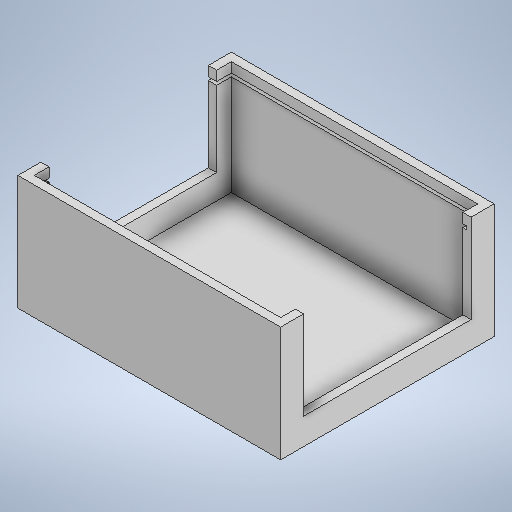
# Autodesk Inventor part: 3 Pzem test
Saved by Autodesk Inventor 2025.3 (Build 293356000, 356)
## iProperties
Created: 2026-02-05
Part Number: 3 Pzem test
Material: Generic
Document SubType Name: Modeling
Designer: Maulana
Density: 1 g/cm^3
Appearance: Default
Author: Maulana
Autodesk Inventor part; units mm, degrees
ref_plane "YZ Plane" through (0, 0, 0) normal (1, 0, 0) x (0, 1, 0)
ref_plane "XZ Plane" through (0, 0, 0) normal (0, 1, 0) x (-1, 0, 0)
sketch "Sketch1" plane through (0, 0, 0) normal (0, 1, 0) x (-1, 0, 0)
  line L0 (37.5, 30) -> (-37.5, 30)
  line L1 (-37.5, 30) -> (-37.5, -30)
  line L2 (-37.5, -30) -> (37.5, -30)
  line L3 (37.5, -30) -> (37.5, 30)
  line L4 (37.5, 30) -> (-37.5, -30) construction
  line L5 (-37.5, 30) -> (37.5, -30) construction
  line L6 (38, 30.5) -> (-38, 30.5)
  line L7 (-38, 30.5) -> (-38, -30.5)
  line L8 (-38, -30.5) -> (38, -30.5)
  line L9 (38, -30.5) -> (38, 30.5)
  line L10 (38, 30.5) -> (-38, -30.5) construction
  line L11 (-38, 30.5) -> (38, -30.5) construction
  point P0 (0, 0)
  dimension "d0" = 75
  dimension "d1" = 60
  dimension "d2" = 76
  dimension "d3" = 61
  constraints: 24 end point, 4 midpoint, 4 parallel, 2 horizontal, 2 perpendicular
  measures "d0" distance of L2.end L1.end
  measures "d1" distance of L1.end L0.end
  measures "d2" distance of L8.end L7.end
  measures "d3" distance of L7.end L6.end
extrude "Extrusion1" add sketch "Sketch1" along normal blind 35
sketch "Sketch2" plane through (0, 0, 0) normal (0, -1, 0) x (1, 0, 0)
  line L0 (37.5, -30) -> (37.5, 30) projected
  line L1 (-37.5, 30) -> (37.5, 30)
  line L2 (37.5, 30) -> (37.5, -30)
  line L3 (37.5, -30) -> (-37.5, -30)
  line L4 (-37.5, -30) -> (-37.5, 30)
  line L5 (-37.5, 30) -> (37.5, -30) construction
  line L6 (37.5, 30) -> (-37.5, -30) construction
  point P0 (0, 0)
  constraints: 12 end point, 2 midpoint, 2 parallel, 1 horizontal, 1 perpendicular
extrude "Extrusion2" add sketch "Sketch2" against normal blind 0.5
sketch "Sketch4" plane through (-38, 0, -30.5) normal (-1, 0, 0) x (0, 0, 1)
  line L0 (61, 35) -> (0, 35) projected
  line L1 (0, 35) -> (5, 35)
  line L2 (61, 35) -> (56, 35)
  line L3 (30.5, 0) -> (30.5, 8)
  line L4 (5, 35) -> (56, 35)
  line L5 (56, 35) -> (56, 13)
  line L6 (56, 13) -> (5, 13)
  line L7 (5, 13) -> (5, 35)
  line L8 (5, 35) -> (56, 35)
  line L9 (56, 35) -> (56, 8)
  line L10 (56, 8) -> (5, 8)
  line L11 (5, 8) -> (5, 35)
  point P0 (5, 13)
  dimension "d8" = 5
  dimension "d9" = 5
  dimension "d10" = 8
  constraints: 22 end point, 4 parallel, 2 horizontal, 2 perpendicular, 2 point on line, 1 vertical
  measures "d8" distance of L0.end L1.end
  measures "d9" distance of L0.start L2.end
  measures "d10" distance of L3.start L3.end
extrude "Extrusion3" cut sketch "Sketch4" against normal blind 30
sketch "Sketch6" plane through (38, 0, -30.5) normal (0, 0, -1) x (-1, 0, 0)
  line L0 (0, 0) -> (0, 35) projected
  line L1 (0, 0) -> (76, 0) projected
  line L2 (0, 35) -> (76, 35)
  line L3 (76, 35) -> (76, 0)
  line L4 (76, 0) -> (0, 0)
  line L5 (0, 0) -> (0, 35)
  point P0 (38, 0)
  constraints: 8 end point, 2 parallel, 1 horizontal, 1 perpendicular
extrude "Extrusion4" add sketch "Sketch6" along normal blind 2
sketch "Sketch7" plane through (-38, 0, 30.5) normal (0, 0, 1) x (1, 0, 0)
  line L0 (76, 0) -> (76, 35) projected
  line L1 (0, 0) -> (0, 35) projected
  line L2 (76, 35) -> (0, 35)
  line L3 (0, 35) -> (0, 0)
  line L4 (0, 0) -> (76, 0)
  line L5 (76, 0) -> (76, 35)
  point P0 (38, 0)
  point P1 (0, 35)
  constraints: 8 end point, 2 parallel, 1 horizontal, 1 perpendicular
extrude "Extrusion5" add sketch "Sketch7" along normal blind 2
sketch "Sketch8" plane through (-38, 13, -25.5) normal (-1, 0, 0) x (0, 0, 1)
  line L0 (0, 22) -> (-7, 22) projected
  line L1 (58, -13) -> (-7, -13) projected
  line L2 (-7, 22) -> (58, 22)
  line L3 (58, 22) -> (58, -13)
  line L4 (58, -13) -> (-7, -13)
  line L5 (-7, -13) -> (-7, 22)
  point P0 (25.5, -13)
  point P1 (0, 22)
  point P2 (-7, -13)
  constraints: 8 end point, 2 parallel, 1 horizontal, 1 perpendicular
extrude "Extrusion6" add sketch "Sketch8" along normal blind 2
sketch "Sketch10" plane through (38, 0, -32.5) normal (1, 0, 0) x (0, 0, -1)
  line L0 (-65, 35) -> (0, 35) projected
  line L1 (0, 0) -> (-65, 0) projected
  line L2 (0, 35) -> (-65, 35)
  line L3 (-65, 35) -> (-65, 0)
  line L4 (-65, 0) -> (0, 0)
  line L5 (0, 0) -> (0, 35)
  point P0 (-32.5, 0)
  point P1 (-7, 35)
  point P2 (-7, 35)
  constraints: 8 end point, 2 parallel, 1 horizontal, 1 perpendicular
extrude "Extrusion8" add sketch "Sketch10" along normal blind 2
sketch "Sketch12" plane through (-40, 13, -25.5) normal (-1, 0, 0) x (0, 0, 1)
  line L0 (0, 22) -> (0, -5) projected
  line L1 (0, -5) -> (51, -5) projected
  line L2 (0, 22) -> (51, 22)
  line L3 (51, 22) -> (51, -5)
  line L4 (51, -5) -> (0, -5)
  line L5 (0, -5) -> (0, 22)
  point P0 (25.5, -13)
  constraints: 8 end point, 2 parallel, 1 horizontal, 1 perpendicular
extrude "Extrusion9" cut sketch "Sketch12" against normal blind 30
ref_plane "Work Plane2" through (0, 13, -25.5) normal (-1, 0, 0) x (0, 0, 1)
mirror "Mirror3" about plane through (0, 13, -25.5) normal (-1, 0, 0) of "Extrusion3", "Extrusion9"
sketch "Sketch13" plane through (-40, 13, -25.5) normal (-1, 0, 0) x (0, 0, 1)
  line L0 (0, 22) -> (0, -5) projected
  line L1 (0, 22) -> (0, 18)
  line L2 (51, -5) -> (51, 22) projected
  line L3 (51, 22) -> (51, 18)
  line L4 (-7, 22) -> (-7, -13) projected
  line L5 (-7, 18) -> (-5.5, 18)
  line L6 (-7, 18) -> (-5.5, 18) construction
  line L7 (51, 22) -> (51, 18)
  line L8 (58, -13) -> (58, 22) projected
  line L9 (58, 18) -> (56.5, 18)
  line L10 (-5.5, 18) -> (56.5, 18)
  line L11 (56.5, 18) -> (56.5, 19)
  line L12 (56.5, 19) -> (-5.5, 19)
  line L13 (-5.5, 19) -> (-5.5, 18)
  point P0 (25.5, -13)
  dimension "d25" = 4
  dimension "d26" = 1.5
  dimension "d27" = 0
  dimension "d28" = 4
  dimension "d29" = 1.5
  dimension "d30" = 1
  constraints: 20 end point, 4 point on line, 3 equal length, 3 horizontal, 2 perpendicular, 1 collinear
  measures "d25" distance of L0.start L1.end
  measures "d26" distance of L5.start L5.end
  measures "d27" distance between parallel lines of L5 L6
  measures "d28" distance of L2.end L3.end
  measures "d29" distance of L9.start L9.end
  measures "d30" distance of L11.end L10.end
extrude "Extrusion10" cut sketch "Sketch13" against normal blind 78.5
body "Solid1"
